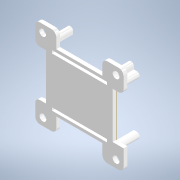
# Autodesk Inventor part: cover
Saved by Autodesk Inventor 2020 (Build 240168000, 168)
## iProperties
Created: 2019-06-14
Part Number: cover
Material: ABS Plastic
Document SubType Name: Modeling
Designer: amirt
Density: 1.06 g/cm^3
Appearance: Smooth - White
Author: amirt
Autodesk Inventor part; units mm, degrees
ref_plane "YZ Plane" through (0, 0, 0) normal (1, 0, 0) x (0, 1, 0)
ref_plane "XZ Plane" through (0, 0, 0) normal (0, 1, 0) x (-1, 0, 0)
ref_plane "XY Plane" through (0, 0, 0) normal (0, 0, 1) x (1, 0, 0)
ref_plane "Work Plane1" through (1.3068, 17.1014, 0) normal (0, 0, 1) x (1, 0, 0)
sketch "Sketch2" plane through (1.3068, 17.1014, 0) normal (0, 0, 1) x (1, 0, 0)
  line L0 (-22, -19.25) -> (-22, 19.25)
  line L1 (-22, 19.25) -> (22, 19.25)
  line L2 (22, -19.25) -> (-22, -19.25)
  line L3 (-22, 19.25) -> (22, 19.25)
  line L4 (22, 19.25) -> (22, -19.25)
  line L5 (-22, 19.25) -> (22, 19.25)
  line L6 (-22, 19.25) -> (-18.19, 19.25)
  line L7 (-22, 15.44) -> (-22, 19.25)
  line L8 (-22, -19.25) -> (-18.19, -19.25)
  line L9 (22, -19.25) -> (18.19, -19.25)
  line L10 (22, -15.44) -> (22, -19.25)
  line L11 (22, 15.44) -> (22, 19.25)
  line L12 (22, 19.25) -> (18.19, 19.25)
  line L13 (18.19, 17.345) -> (-18.19, 17.345)
  line L14 (-18.19, 17.345) -> (-18.19, 15.44)
  line L15 (-18.19, 15.44) -> (18.19, 15.44)
  line L16 (18.19, 15.44) -> (18.19, 17.345)
  line L17 (18.19, -17.345) -> (-18.19, -17.345)
  line L18 (-18.19, -17.345) -> (-18.19, -15.44)
  line L19 (-18.19, -15.44) -> (18.19, -15.44)
  line L20 (18.19, -15.44) -> (18.19, -17.345)
  circle A0 centre (-24.1175, -24.3391) radius 2.25 projected
  circle A1 centre (-24.2491, 24.2487) radius 2.25 projected
  circle A2 centre (24.2419, 24.2487) radius 2.25 projected
  circle A3 centre (24.2419, -24.2423) radius 2.25 projected
  line L21 (15.2616, -22.247) -> (15.2616, -26.057) projected
  arc A4 (15.2616, -26.057) -> (18.4366, -29.232) centre (18.4366, -26.057) ccw projected
  line L22 (18.4366, -29.232) -> (26.0566, -29.232) projected
  arc A5 (26.0566, -29.232) -> (29.2316, -26.057) centre (26.0566, -26.057) ccw projected
  line L23 (29.2316, -26.057) -> (29.2316, -15.262) projected
  line L24 (29.2316, -15.262) -> (18.3723, -15.262) projected
  line L25 (18.3723, 15.2684) -> (26.0566, 15.2684) projected
  arc A6 (26.0566, 15.2684) -> (29.2316, 18.4434) centre (26.0566, 18.4434) ccw projected
  line L26 (29.2316, 18.4434) -> (29.2316, 26.0634) projected
  arc A7 (29.2316, 26.0634) -> (26.0566, 29.2384) centre (26.0566, 26.0634) ccw projected
  line L27 (26.0566, 29.2384) -> (18.4366, 29.2384) projected
  line L28 (15.2616, 26.0634) -> (15.2616, 22.2534) projected
  arc A8 (18.4366, 29.2384) -> (15.2616, 26.0634) centre (18.4366, 26.0634) ccw projected
  line L29 (-26.0638, 15.2684) -> (-15.2688, 15.2684) projected
  arc A9 (-29.2388, 18.4434) -> (-26.0638, 15.2684) centre (-26.0638, 18.4434) ccw projected
  line L30 (-29.2388, 26.0634) -> (-29.2388, 18.4434) projected
  arc A10 (-26.0638, 29.2384) -> (-29.2388, 26.0634) centre (-26.0638, 26.0634) ccw projected
  line L31 (-18.4438, 29.2384) -> (-26.0638, 29.2384) projected
  arc A11 (-15.2688, 26.0634) -> (-18.4438, 29.2384) centre (-18.4438, 26.0634) ccw projected
  line L32 (-15.2688, 22.2534) -> (-15.2688, 26.0634) projected
  line L33 (-15.2688, -26.057) -> (-15.2688, -22.247) projected
  arc A12 (-18.4438, -29.232) -> (-15.2688, -26.057) centre (-18.4438, -26.057) ccw projected
  line L34 (-26.0638, -29.232) -> (-18.4438, -29.232) projected
  arc A13 (-29.2388, -26.057) -> (-26.0638, -29.232) centre (-26.0638, -26.057) ccw projected
  line L35 (-29.2388, -18.437) -> (-29.2388, -26.057) projected
  arc A14 (-26.0638, -15.262) -> (-29.2388, -18.437) centre (-26.0638, -18.437) ccw projected
  line L36 (-15.2688, -15.262) -> (-26.0638, -15.262) projected
  line L37 (-15.2688, -22.247) -> (-15.2688, -19.25)
  line L38 (15.2616, -22.247) -> (15.2616, -19.25)
  line L39 (15.2616, 22.2534) -> (15.2616, 19.25)
  line L40 (-15.2688, 22.2534) -> (-15.2688, 19.25)
  point P0 (-1.3068, -17.1014)
  point P1 (0, 0)
  point P2 (22, -15.262)
  point P3 (18.19, -19.25)
  point P4 (15.2616, 19.25)
  point P5 (22, 15.2684)
  point P6 (-22, 15.2684)
  point P7 (-22, -15.262)
  constraints: 50 end point, 8 point on line, 6 horizontal, 4 parallel, 4 perpendicular
extrude "Extrusion2" add sketch "Sketch2" along normal blind 2.54
sketch "Sketch4" plane through (1.3068, 17.1014, 0) normal (0, 0, -1) x (-1, 0, 0)
  line L0 (22, 21.155) -> (22, 19.25) projected
  arc A0 (22, 21.155) -> (18.19, 21.155) centre (20.095, 21.155) ccw projected
  line L1 (18.19, 19.25) -> (18.19, 21.155) projected
  line L2 (22, 19.25) -> (23.905, 19.25) projected
  arc A1 (23.905, 15.44) -> (23.905, 19.25) centre (23.905, 17.345) ccw projected
  line L3 (23.905, 15.44) -> (22, 15.44) projected
  line L4 (-23.905, 19.25) -> (-22, 19.25) projected
  arc A2 (-23.905, 19.25) -> (-23.905, 15.44) centre (-23.905, 17.345) ccw projected
  line L5 (-22, 15.44) -> (-23.905, 15.44) projected
  line L6 (-22, 19.25) -> (-22, 21.155) projected
  arc A3 (-18.19, 21.155) -> (-22, 21.155) centre (-20.095, 21.155) ccw projected
  line L7 (-18.19, 21.155) -> (-18.19, 19.25) projected
  line L8 (-23.905, -15.44) -> (-22, -15.44) projected
  arc A4 (-23.905, -15.44) -> (-23.905, -19.25) centre (-23.905, -17.345) ccw projected
  line L9 (-22, -19.25) -> (-23.905, -19.25) projected
  line L10 (-22, -21.155) -> (-22, -19.25) projected
  arc A5 (-22, -21.155) -> (-18.19, -21.155) centre (-20.095, -21.155) ccw projected
  line L11 (-18.19, -19.25) -> (-18.19, -21.155) projected
  line L12 (18.19, -21.155) -> (18.19, -19.25) projected
  arc A6 (18.19, -21.155) -> (22, -21.155) centre (20.095, -21.155) ccw projected
  line L13 (22, -19.25) -> (22, -21.155) projected
  line L14 (23.905, -19.25) -> (22, -19.25) projected
  line L15 (22, -15.44) -> (23.905, -15.44) projected
  arc A7 (23.905, -19.25) -> (23.905, -15.44) centre (23.905, -17.345) ccw projected
  line L16 (22, -15.44) -> (22, -19.25)
  line L17 (18.19, -19.25) -> (22, -19.25)
  line L18 (-22, -19.25) -> (-18.19, -19.25)
  line L19 (-22, -15.44) -> (-22, -19.25)
  line L20 (-22, 19.25) -> (-22, 15.44)
  line L21 (-22, 19.25) -> (-18.19, 19.25)
  line L22 (18.19, 19.25) -> (22, 19.25)
  line L23 (22, 21.155) -> (22, 19.25) projected
  line L24 (22, 15.44) -> (22, 19.25)
  point P0 (1.3068, -17.1014)
  constraints: 16 end point, 3 perpendicular, 2 collinear, 2 vertical, 1 horizontal
extrude "Extrusion3" add sketch "Sketch4" along normal blind 11.545
body "Solid1"
